SceneCube Light Stand (Autodesk Fusion 360 design; units mm, degrees)
Autodesk Fusion 360 part; units mm, degrees
sketch "Sketch2" plane through (0, 0, 0) normal (0, 1, 0) x (1, 0, 0)
  circle A0 centre (0, 0) radius 6.75
  circle A1 centre (0, 0) radius 4.25
  line L0 (-3.2862, 6.75) -> (3.2138, 6.75)
  line L1 (3.2138, 6.75) -> (3.2138, 3.75)
  line L2 (3.2138, 3.75) -> (-3.2862, 3.75)
  line L3 (-3.2862, 3.75) -> (-3.2862, 6.75)
  circle A2 centre (0, -4) radius 5.75
  dimension "d1" = 13.5
  dimension "d2" = 8.5
  dimension "d3" = 6.5
  dimension "d4" = 3
  dimension "d5" = 11.5
  constraint coincident A0.centre A1.centre
  constraint concentric A0 A1
  constraint horizontal L0
  constraint vertical L1
  constraint horizontal L2
  constraint vertical L3
  constraint tangent A0 L0
  measures "d1" diameter of A0
  measures "d2" diameter of A1
  measures "d3" distance of L0.start L0.end
  measures "d4" distance of L0.start L2.end
  measures "d5" diameter of A2
extrude "Extrude1" add sketch "Sketch2" along normal blind 3.5 contours A0 A1 L1 L2 A2 | A0 A1 A2 | A0 A1 L2 L3 A2 | A1 L2 A2
sketch "Sketch4" plane through (0, 0, 0) normal (1, 0, 0) x (0, 0, -1)
  line L0 (-0.5599, 30.5) -> (0.5599, 30.5)
  line L1 (0.5599, 30.5) -> (0.5599, 13.5)
  line L2 (0.5599, 13.5) -> (-0.5599, 13.5)
  line L3 (-0.5599, 13.5) -> (-0.5599, 30.5)
  line L4 (-0.5599, 30.5) -> (0.5599, 13.5) construction
  line L5 (0.5599, 30.5) -> (-0.5599, 13.5) construction
  line L6 (5.9358, 3.5) -> (-6.75, 3.5)
  line L7 (3.75, 10) -> (1.25, 10)
  line L8 (1.25, 10) -> (1.25, 0)
  line L9 (1.25, 0) -> (3.75, 0)
  line L10 (3.75, 0) -> (3.75, 10)
  line L11 (3.75, 10) -> (0.5599, 13.5)
  line L12 (-0.5599, 13.5) -> (1.25, 10)
  point P0 (0, 22)
  dimension "d8" = 17
  dimension "d9" = 18.5
  dimension "d10" = 2.5
  dimension "d11" = 1.25
  dimension "d12" = 10
  constraint perpendicular L0 L1
  constraint parallel L0 L2
  constraint parallel L1 L3
  constraint horizontal L0
  constraint coincident L4 P0
  constraint coincident L5 P0
  constraint vertical origin P0
  constraint horizontal L7
  constraint vertical L8
  constraint horizontal L9
  constraint vertical L10
  constraint coincident origin L9
  measures "d8" distance of L0.end L1.end
  measures "d9" distance of P0 L6
  measures "d10" distance of L8.end L9.end
  measures "d11" distance of origin L8
  measures "d12" distance of L7.start L9.end
extrude "Extrude2" add sketch "Sketch4" along normal mid plane 8
